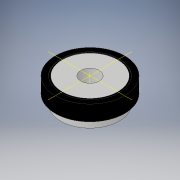
# Autodesk Inventor part: BT602_trajan20_21
Saved by Autodesk Inventor 2022.2 (Build 262287000, 287)
## iProperties
Company: HTBLA Kaindorf
RuleStatus: InUse
Created: 2022-09-09
Part Number: BT602_trajan20_21
Project: Zeichenmaschine_v2
Material: Generisch
Description: rollte
Document SubType Name: Modeling
Designer: trajan20
Density: 1 g/cm^3
Appearance: Vorgabe
Mass: 20.8701 g
Surface Area: 57.6126 cm^2
Volume: 20.8701 cm^3
AfterDocNew0: iProperties-Editor_aufrufen
Author: jan
Keywords: 2021
Autodesk Inventor part; units mm, degrees
ref_plane "YZ Plane" through (0, 0, 0) normal (1, 0, 0) x (0, 1, 0)
ref_plane "XZ Plane" through (0, 0, 0) normal (0, 1, 0) x (-1, 0, 0)
ref_plane "XY Plane" through (0, 0, 0) normal (0, 0, 1) x (1, 0, 0)
sketch "Skizze3" plane through (0, 0, 0) normal (0, 1, 0) x (-1, 0, 0)
  line L0 (0, 0) -> (0, -18.1445)
  line L1 (6, 0) -> (6, -16)
  line L2 (6, -16) -> (19, -16)
  line L3 (19, -16) -> (19, -10)
  line L4 (19, -10) -> (22.5, -10)
  line L5 (22.5, -10) -> (22.5, 0)
  line L6 (22.5, 0) -> (19, 0)
  line L7 (19, 0) -> (19, -0.5)
  line L8 (19, -0.5) -> (18, 0)
  line L9 (18, 0) -> (6, 0)
  point P0 (19, -0.25)
  dimension "d4" = 16
  dimension "d5" = 10
  dimension "d6" = 12
  dimension "d7" = 38
  dimension "d8" = 45
  dimension "d9" = 1
  dimension "d10" = 0.5
  constraints: 20 end point, 4 perpendicular, 3 point on line, 2 horizontal, 2 vertical, 1 collinear, 1 midpoint
  measures "d4" distance between parallel lines of L2 L9
  measures "d5" distance between parallel lines of L6 L4
  measures "d6" diameter of L1 L0
  measures "d7" diameter of L3 L0
  measures "d8" diameter of L5 L0
  measures "d9" distance from line of L7 L8.end
  measures "d10" distance of L6.end L7.end
revolve "Umdrehung1" add sketch "Skizze3" angle 360 about axis through (0, 0, 0) along (0, 0, -1)
